Vorhangkappe_v3 (Autodesk Fusion 360 design; units mm, degrees)
Autodesk Fusion 360 part; units mm, degrees
sketch "Skizze1" plane through (0, 0, 0) normal (0, 1, 0) x (1, 0, 0)
  line L0 (0, 0) -> (19, 0)
  line L1 (19, 0) -> (18.5, -18)
  line L2 (18.5, -18) -> (0.5, -18)
  line L3 (0.5, -18) -> (0, 0)
  line L4 (1.5, -1.5) -> (17.5, -1.5)
  line L5 (17.5, -1.5) -> (17, -16.5)
  line L6 (17, -16.5) -> (2, -16.5)
  line L7 (2, -16.5) -> (1.5, -1.5)
  dimension "d2" = 19
  dimension "d3" = 16
  dimension "d20" = 18
  dimension "d21" = 15
  dimension "d22" = 0.5
  dimension "d23" = 1.5
  dimension "d24" = 2
  dimension "d25" = 18
  dimension "d26" = 15
  dimension "d27" = 1.5
  constraint horizontal L0
  constraint horizontal L2
  constraint coincident L0.start L3.end
  constraint horizontal L4
  constraint horizontal L6
  measures "d2" distance of L0.start L0.end
  measures "d3" distance of L4.start L4.end
  measures "d20" distance of L1.end L2.end
  measures "d21" distance of L5.end L6.end
  measures "d22" horizontal distance of L0.start L2.end
  measures "d23" horizontal distance of L0.start L4.start
  measures "d24" horizontal distance of L0.start L6.end
  measures "d25" vertical distance of L0.start L2.end
  measures "d26" vertical distance of L4.start L6.end
  measures "d27" vertical distance of L0.start L4.start
extrude "Extrusion1" add sketch "Skizze1" along normal blind 15
move_face "Fläche verschieben1" by (0.15, 0, 0) 1 faces at (1.8333, 5, 11.5)
move_face "Fläche verschieben2" by (0, 0, 0.15) 1 faces at (6.9333, 5, 1.5)
move_face "Fläche verschieben3" by (-0.15, 0, 0) 1 faces at (17.33, 5, 6.6)
move_face "Fläche verschieben4" by (0, 0, -0.15) 1 faces at (11.95, 5, 16.5)
move_face "Fläche verschieben5" to x (1, 0, 0) y (0, 0.997801, -0.066274) z (0, 0.066274, 0.997801) at (0, -0.1094, 0.0036) 1 faces at (6.885, 5, 1.65)
move_face "Fläche verschieben6" to x (0.997804, 0.066237, 0.000073) y (-0.066237, 0.997801, 0.002208) z (0.000073, -0.002208, 0.999998) at (0.0035, -0.106, -0.0001) 1 faces at (1.8073, 10, 6.2179)
move_face "Fläche verschieben7" to x (1, 0, 0) y (0, 0.99945, 0.033155) z (0, -0.033155, 0.99945) at (0, 0.5421, 0.009) 1 faces at (6.716, 10, 16.35)
move_face "Fläche verschieben8" to x (0.999451, -0.033137, -0.000018) y (0.033137, 0.99945, 0.001105) z (-0.000018, -0.001105, 0.999999) at (0.0096, 0.5766, 0.0003) 1 faces at (17.1872, 10, 6.3838)
move_face "Fläche verschieben9" to x (1, 0, 0) y (0, 0.99945, 0.033155) z (0, -0.033155, 0.99945) at (0, 0.0547, 0.0009) 1 faces at (6.7187, 10, 0.9858)
move_face "Fläche verschieben10" to x (0.999451, -0.033137, 0.000018) y (0.033137, 0.99945, -0.001105) z (0.000018, 0.001105, 0.999999) at (0.0009, 0.053, 0) 1 faces at (1.1538, 10, 6.55)
extrude "Extrude2" add sketch "Skizze1" against normal blind 1 contours L0 L1 L2 L3 | L4 L5 L6 L7
fillet "Abrundung1" radius 0.5 6 faces at (17.5136, 10, 6.55) (12.115, 10, 1.3183) (6.3333, 4.3333, 0) (6.7135, 15, 0.3841) (0.3333, 4.3333, 12) (12.5, 4.3333, 18)
fillet "Abrundung1" radius 0.5 3 edges at (1.9044, 7.5, 16.5988) (9.5, 0, 16.35) (1.9, 0, 9)
fillet "Abrundung1" radius 0.5 1 edges at (18.75, -1, 9)
equation "d22 = ( d2 - d20 ) / 2"
equation "d23 = ( d2 - d3 ) / 2"
equation "d24 = ( d2 - d21 ) / 2"
equation "d27 = ( d25 - d26 ) / 2"
